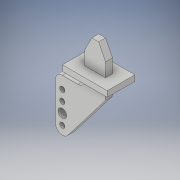
# Autodesk Inventor part: Control Horn
Saved by Autodesk Inventor 2019 (Build 230136000, 136)
## iProperties
Created: 2021-08-25
Part Number: Control Horn
Material: Generic
Document SubType Name: Modeling
Designer: HP
Density: 1 g/cm^3
Appearance: Default
Author: HP
Autodesk Inventor part; units mm, degrees
ref_plane "YZ Plane" through (0, 0, 0) normal (1, 0, 0) x (0, 1, 0)
ref_plane "XZ Plane" through (0, 0, 0) normal (0, 1, 0) x (-1, 0, 0)
ref_plane "XY Plane" through (0, 0, 0) normal (0, 0, 1) x (1, 0, 0)
sketch "Sketch1" plane through (0, 0, 0) normal (0, 0, 1) x (1, 0, 0)
  line L0 (0, 0) -> (0, -1.65)
  line L1 (0, -1.65) -> (13, -1.65)
  line L2 (13, -1.65) -> (13, 0)
  line L3 (13, 0) -> (0, 0)
  dimension "d1" = 1.65
  dimension "d2" = 13
  constraints: 8 end point, 2 perpendicular, 1 horizontal, 1 vertical
  measures "d1" distance of L0.start L0.end
  measures "d2" distance of L0.end L1.end
extrude "Extrusion1" add sketch "Sketch1" along normal blind 8
sketch "Sketch3" plane through (0, 0, 0) normal (0, 1, 0) x (1, 0, 0)
  line L0 (0, 0) -> (13, 0) projected
  line L1 (0, -8) -> (13, -8) projected
  line L2 (0, 0) -> (0, -8) projected
  line L3 (0, 0) -> (0, -3)
  line L4 (0, -8) -> (0, -5)
  line L5 (13, 0) -> (13, -3)
  line L6 (13, 0) -> (13, -8) projected
  line L7 (13, -8) -> (13, -5)
  line L8 (3.5, -3) -> (9.5, -3)
  line L9 (9.5, -3) -> (9.5, -5)
  line L10 (9.5, -5) -> (3.5, -5)
  line L11 (3.5, -5) -> (3.5, -3)
  dimension "d9" = 3
  dimension "d10" = 3
  dimension "d13" = 3.5
  dimension "d14" = 3.5
  constraints: 16 end point, 4 point on line, 2 parallel, 1 horizontal, 1 perpendicular
  measures "d9" distance of L0.start L3.end
  measures "d10" distance of L1.start L4.end
  measures "d13" distance of L3.end L8.start
  measures "d14" distance of L7.end L9.end
extrude "Extrusion2" add sketch "Sketch3" along normal blind 8 contours L8 L9 L10 L11
sketch "Sketch4" plane through (0, -1.65, 0) normal (0, -1, 0) x (1, 0, 0)
  line L0 (13, 8) -> (0, 8) projected
  line L1 (13, 0) -> (13, 8) projected
  line L2 (13, 8) -> (13, 5)
  line L3 (13, 5) -> (13, 3)
  line L4 (9.5, 5) -> (3.5, 5) projected
  line L5 (3.5, 5) -> (3.5, 3) projected
  line L6 (3.5, 5) -> (9.5, 5)
  line L7 (9.5, 5) -> (9.5, 3)
  line L8 (9.5, 3) -> (3.5, 3)
  line L9 (3.5, 3) -> (3.5, 5)
  constraints: 12 end point, 2 parallel, 2 point on line, 1 horizontal, 1 perpendicular
extrude "Extrusion3" add sketch "Sketch4" along normal blind 4
sketch "Sketch6" plane through (9.5, -1.65, 3) normal (0, 0, -1) x (-1, 0, 0)
  line L0 (0, -4) -> (6, -4) projected
  line L1 (6, -4) -> (14.5, -4)
  line L2 (14.5, -4) -> (14.5, -19)
  line L3 (14.5, -19) -> (11.5, -19)
  line L4 (11.5, -19) -> (0, -4)
  point P0 (9.5, 1.65)
  dimension "d22" = 8.5
  dimension "d23" = 15
  dimension "d24" = 3
  constraints: 8 end point, 2 horizontal, 1 vertical
  measures "d22" distance of L0.end L1.end
  measures "d23" distance of L1.end L2.end
  measures "d24" distance of L2.end L3.end
extrude "Extrusion4" add sketch "Sketch6" against normal blind 2
sketch "Sketch7" plane through (9.5, -1.65, 3) normal (0, 0, -1) x (-1, 0, 0)
  line L0 (6, -4) -> (14.5, -4) projected
  line L1 (14.5, -19) -> (12.5, -19)
  line L2 (14.5, -19) -> (11.5, -19) projected
  line L3 (12.5, -4) -> (12.5, -6.5)
  line L4 (12.5, -19) -> (12.5, -16.5)
  circle A0 centre (12.5, -16.5) radius 0.75
  line L5 (12.5, -16.5) -> (12.5, -13.5)
  circle A1 centre (12.5, -13.5) radius 1.25
  line L6 (12.5, -13.5) -> (12.5, -10.5)
  circle A2 centre (12.5, -10.5) radius 0.75
  line L7 (12.5, -10.5) -> (12.5, -7.5)
  circle A3 centre (12.5, -7.5) radius 0.75
  point P0 (9.5, 1.65)
  dimension "d31" = 2
  dimension "d45" = 2.5
  dimension "d46" = 2.5
  dimension "d47" = 1.5
  dimension "d48" = 3
  dimension "d49" = 2.5
  dimension "d50" = 3
  dimension "d51" = 1.5
  dimension "d52" = 3
  dimension "d53" = 1.5
  constraints: 12 end point, 4 centre point, 4 coincident, 3 vertical, 2 point on line, 1 perpendicular
  measures "d31" distance of L1.start L1.end
  measures "d45" distance of L3.start L3.end
  measures "d46" distance of L1.end L4.end
  measures "d47" diameter of A0
  measures "d48" distance of L5.start L5.end
  measures "d49" diameter of A1
  measures "d50" distance of L6.start L6.end
  measures "d51" diameter of A2
  measures "d52" distance of L7.start L7.end
  measures "d53" diameter of A3
fillet "Fillet1" radius 2 1 edges at (3.5, -5.65, 4)
fillet "Fillet2" radius 2 2 edges at (-2, -20.65, 4) (-5, -20.65, 4)
fillet "Fillet3" radius 2 1 edges at (-5, -5.65, 4)
extrude "Extrusion6" cut sketch "Sketch7" against normal blind 2
sketch "Sketch8" plane through (9.5, -1.65, 3) normal (0, 0, -1) x (-1, 0, 0)
  line L0 (0, 1.65) -> (0, 9.65) projected
  line L1 (0, 1.65) -> (0, 5.65)
  line L2 (0, 9.65) -> (2, 9.65)
  line L3 (6, 9.65) -> (4, 9.65)
  line L4 (6, 9.65) -> (0, 9.65) projected
  line L5 (-3.5, 1.65) -> (9.5, 1.65) projected
  line L6 (6, 1.65) -> (6, 5.65)
  line L7 (0, 9.65) -> (2, 9.65)
  line L8 (2, 9.65) -> (0, 5.65)
  line L9 (0, 5.65) -> (0, 9.65)
  line L10 (4, 9.65) -> (6, 5.65)
  line L11 (6, 1.65) -> (6, 9.65) projected
  line L12 (6, 9.65) -> (6, 5.65)
  line L13 (4, 9.65) -> (6, 9.65)
  dimension "d59" = 4
  dimension "d60" = 2
  dimension "d61" = 2
  constraints: 20 end point, 4 collinear, 2 point on line, 1 horizontal, 1 midpoint, 1 vertical
  measures "d59" distance of L0.start L1.end
  measures "d60" distance of L0.end L2.end
  measures "d61" distance of L3.start L3.end
extrude "Extrusion7" cut sketch "Sketch8" against normal blind 10 contours L0 L2 L8 | L10 L3 L11
body "Solid1"
